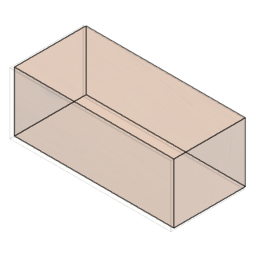
Mortise and tenon joint (Autodesk Fusion 360 design; units mm, degrees)
Autodesk Fusion 360 part; units mm, degrees
sketch "Contact Patch" plane through (0, 0, 0) normal (0, 0, 1) x (1, 0, 0)
  line L0 (50, -20) -> (-50, -20)
  line L1 (-50, -20) -> (-50, 20)
  line L2 (-50, 20) -> (50, 20)
  line L3 (50, 20) -> (50, -20)
  line L4 (50, -20) -> (-50, 20) construction
  line L5 (-50, -20) -> (50, 20) construction
  dimension "d3" = 100
  dimension "d4" = 40
  constraint horizontal L0
  constraint perpendicular L0 L1
  constraint parallel L0 L2
  constraint parallel L1 L3
  constraint coincident L4 origin
  constraint coincident L5 origin
  measures "d3" distance of L0.start L0.end
  measures "d4" distance of L0 L2
sketch "Tenon" plane through (0, 0, 0) normal (0, 0, 1) x (1, 0, 0)
  line L0 (40, -15) -> (-40, -15)
  line L1 (-40, -15) -> (-40, 15)
  line L2 (-40, 15) -> (40, 15)
  line L3 (40, 15) -> (40, -15)
  line L4 (40, -15) -> (-40, 15) construction
  line L5 (-40, -15) -> (40, 15) construction
  line L6 (-50, -20) -> (-50, 20)
  line L7 (-50, 20) -> (50, 20)
  dimension "d7" = 10
  dimension "d8" = 5
  constraint horizontal L0
  constraint perpendicular L0 L1
  constraint parallel L0 L2
  constraint parallel L1 L3
  constraint coincident L4 origin
  constraint coincident L5 origin
  measures "d7" distance of L1 L6
  measures "d8" distance of L2 L7
extrude "Extrude1" add sketch "Tenon" along normal blind 35 makes body 1
move_face "OffsetFaces1" offset 1 1 faces at (13.3333, 5, 0) on bodies 1
sketch "Sketch3" plane through (0, 0, 0) normal (0, 0, 1) x (1, 0, 0)
  line L0 (40, 15) -> (-40, 15)
  line L1 (-40, 15) -> (-40, -15)
  line L2 (-40, -15) -> (40, -15)
  line L3 (40, -15) -> (40, 15)
  line L4 (-40.5, -15.5) -> (40.5, -15.5)
  line L5 (40.5, -15.5) -> (40.5, 15.5)
  line L6 (40.5, 15.5) -> (-40.5, 15.5)
  line L7 (-40.5, 15.5) -> (-40.5, -15.5)
  dimension "d14" = 0.5
extrude "Extrude2" add sketch "Sketch3" along normal blind 37 separate body contours L0 L1 L2 L3 | L4 L5 L6 L7 makes body 2
equation "Length = 100 mm"
equation "Width = 40 mm"
equation "d3 = Length"
equation "d4 = Width"
equation "EndOffset = 10 mm"
equation "SideOffset = 5 mm"
equation "d7 = EndOffset"
equation "d8 = SideOffset"
equation "Tenon_length = 35 mm"
equation "d10 = Tenon_length"
equation "Clearance = 0.5 mm"
equation "d14 = Clearance"
equation "Bottom_gap = 2 mm"
equation "Mortise_length = Tenon_length + Bottom_gap"
equation "d17 = Mortise_length"
named bodies: "Tenon", "Mortise"
